Autodesk Fusion 360 part; units mm, degrees
(part 4 of 4)
extrude "Extrude2" cut sketch "IronHandPCBPlate" along normal blind 1.2 contours L457 L479 L536 L538 L540 L541 L542 L543 bodies 1
extrude "Extrude3" add sketch "Sketch3" along normal blind 1 separate body contours A4 | L212 L490 L491 L492 L495 | L212 L486 L492 L496 | L212 L484 L485 L486 L489 L495 L496 | L212 L483 L484 L487 L489 L494 L495 | L212 L467 L486 L492 | L212 L213 L214 L218 L464 L466 L467 L468 L477 L478 L479 L481 L490 L491 L492 L499 L518 | L486 L492 L496 L511 | L485 L486 L496 L497 L505 | L212 L213 L487 L490 L494 | L482 L483 L484 L485 L502 | L467 L486 L492 L511 | L492 L493 L497 L498 L505 L509 L511 | L483 L487 L494 L497 L503 | L213 L487 L490 L493 L494 L497 L498 L503 | L467 L492 L509 L511 | L482 L497 L502 L505 L517 | L493 L497 L498 L505 L509 L517 | L493 L498 L501 L505 L509 L515 | L467 L501 L508 L509 L515 | L482 L497 L502 L503 L517 | L493 L497 L498 L503 L517 | L493 L498 L505 L509 L510 L515 | L213 L493 L498 L499 L500 L503 L504 L506 L507 | L501 L505 L513 L515 | L467 L501 L508 L513 L514 L515 | L493 L498 L503 L504 L510 L513 L515 L516 | L505 L510 L513 L515 | L213 L466 L467 L500 L512 L518 | L501 L505 L507 L513 | L467 L501 L507 L508 L513 | L510 L513 L515 L516 | L504 L505 L507 L510 L513 | L214 L466 L468 L477 L518 L519 L520 L521 | L500 L501 L504 L506 L507 | L467 L501 L507 L512 | A249 | A458 makes body 2
extrude "Extrude4" add sketch "Sketch3" along normal blind 5.5 contours L212 L490 L491 L492 L495 | L212 L486 L492 L496 | L212 L484 L485 L486 L489 L495 L496 | L212 L483 L484 L487 L489 L494 L495 | L486 L492 L496 L511 | L485 L486 L496 L497 L505 | L212 L213 L487 L490 L494 | L492 L493 L497 L498 L505 L509 L511 | L483 L487 L494 L497 L503 | L213 L487 L490 L493 L494 L497 L498 L503 | L467 L492 L509 L511 | L482 L497 L502 L505 L517 | L493 L497 L498 L505 L509 L517 | L493 L498 L501 L505 L509 L515 | L467 L501 L508 L509 L515 | L482 L497 L502 L503 L517 | L493 L497 L498 L503 L517 | L493 L498 L505 L509 L510 L515 | L213 L493 L498 L499 L500 L503 L504 L506 L507 | L501 L505 L513 L515 | L467 L501 L508 L513 L514 L515 | L493 L498 L503 L504 L510 L513 L515 L516 | L505 L510 L513 L515 | L501 L505 L507 L513 | L467 L501 L507 L508 L513 | L510 L513 L515 L516 | L504 L505 L507 L510 L513 | L500 L501 L504 L506 L507 | L467 L501 L507 L512 bodies 2
extrude "Extrude5" cut sketch "Sketch3" against normal blind 3 from surface at 5.5 contours L212 L484 L485 L486 L489 L495 L496 | L212 L483 L484 L487 L489 L494 L495 | L485 L486 L496 L497 L505 | L483 L487 L494 L497 L503 | L482 L497 L502 L505 L517 | L482 L497 L502 L503 L517 bodies 2
extrude "Extrude8" add sketch "Sketch3" along normal blind 4.5 contours L493 L498 L501 L505 L509 L515 | L467 L501 L508 L509 L515 | L493 L498 L505 L509 L510 L515 | L501 L505 L513 L515 | L467 L501 L508 L513 L514 L515 | L493 L498 L503 L504 L510 L513 L515 L516 | L505 L510 L513 L515 | L501 L505 L507 L513 | L467 L501 L507 L508 L513 | L510 L513 L515 L516 | L504 L505 L507 L510 L513 bodies 2
sketch "Sketch4" plane through (0, 0, 7.5) normal (0, 0, 1) x (-1, 0, 0)
  line L0 (37.7668, 220.6) -> (37.7667, 165.6443)
  line L1 (37.7667, 165.6443) -> (61.9431, 165.6443)
  line L2 (61.9431, 165.6443) -> (61.9431, 201.6)
  line L3 (60.9431, 166.6443) -> (38.7668, 166.6443)
  line L4 (38.7667, 166.6443) -> (38.7667, 201.6)
  line L5 (38.7667, 201.6) -> (60.9431, 201.6)
  line L6 (60.9431, 201.6) -> (60.9431, 166.6443)
  line L7 (67.9431, 220.6) -> (37.7668, 220.6)
  line L8 (61.9431, 201.6) -> (67.9431, 201.6)
  line L9 (67.9431, 201.6) -> (67.9431, 220.6)
  line L10 (67.9431, 231.6) -> (64.9431, 231.6) construction
  line L11 (64.9431, 231.6) -> (64.9431, 229.1)
  line L12 (64.9431, 229.1) -> (67.9431, 229.1)
  line L13 (67.9431, 229.1) -> (67.9431, 231.6) construction
  line L14 (67.9431, 229.1) -> (64.9431, 229.1)
  line L15 (64.9431, 229.1) -> (64.9431, 226.1)
  line L16 (64.9431, 226.1) -> (67.9431, 226.1)
  line L17 (67.9431, 226.1) -> (67.9431, 229.1)
  line L18 (38.7667, 166.6443) -> (38.7667, 201.6)
  line L19 (38.7667, 201.6) -> (60.9431, 201.6)
  line L20 (60.9431, 201.6) -> (60.9431, 166.6443)
  line L21 (60.9431, 166.6443) -> (38.7668, 166.6443)
  point P0 (67.9431, 231.6)
  point P1 (67.9431, 231.6)
  dimension "d76" = 3
  dimension "d77" = 2.5
  dimension "d100" = 3
  dimension "d101" = 3
  constraint horizontal L3
  constraint vertical L4
  constraint horizontal L5
  constraint vertical L6
  constraint horizontal L10
  constraint vertical L11
  constraint horizontal L12
  constraint vertical L13
  constraint coincident P1 P0
  constraint horizontal L14
  constraint vertical L15
  constraint horizontal L16
  constraint vertical L17
  measures "d76" distance of P1 L10.end
  measures "d77" distance of P1 L12.end
  measures "d100" distance of L12.end L11.end
  measures "d101" distance of L12.end L16.end
extrude "Extrude6" add sketch "Sketch4" against normal blind 3 separate body contours L3 L4 L5 L6 L18 L19 L20 L21 makes body 3
extrude "Extrude7" cut sketch "Sketch3" along normal blind 2.5 contours L482 L483 L484 L485 L502 | L482 L497 L502 L505 L517 | L493 L497 L498 L505 L509 L517 | L493 L498 L501 L505 L509 L515 | L467 L501 L508 L509 L515 | L493 L498 L505 L509 L510 L515 | L501 L505 L513 L515 | L467 L501 L508 L513 L514 L515 | L505 L510 L513 L515 | L501 L505 L507 L513 | L467 L501 L507 L508 L513 | L504 L505 L507 L510 L513 bodies 2
extrude "Extrude9" cut sketch "Sketch3" along normal blind 3.5 contours L501 L505 L513 L515 | L467 L501 L508 L513 L514 L515 | L505 L510 L513 L515 bodies 2
extrude "Extrude10" add sketch "Sketch4" against normal up to surface (2.5 mm away) from surface at -5 contours L12 L14 L15 L16 L17 bodies 2
sketch "Sketch5" plane through (-67.9431, 0, 0) normal (-1, 0, 0) x (0, -1, 0)
  line L0 (218.7407, 5.5) -> (218.7407, 4.5)
  line L1 (218.7407, 4.5) -> (219.6, 4.5)
  line L2 (219.6, 4.5) -> (219.6, 2)
  line L3 (229.1, 2) -> (231.6, 2)
  line L4 (226.1, 0) -> (229.1, 0)
  line L5 (231.6, 3) -> (220.6, 3)
  line L6 (220.6, 3) -> (220.6, 7.5)
  line L7 (220.6, 7.5) -> (201.6, 7.5)
  line L8 (201.6, 7.5) -> (201.6, 3)
  line L9 (201.6, 3) -> (156.6443, 3)
  line L10 (156.6443, 3) -> (156.6443, 2)
  line L11 (156.6443, 2) -> (202.6, 2)
  line L12 (202.6, 2) -> (202.6, 4.5)
  line L13 (202.6, 4.5) -> (203.6, 4.5)
  line L14 (203.6, 4.5) -> (203.6, 5.5)
  line L15 (203.6, 5.5) -> (218.7407, 5.5)
  line L16 (202.6, 6.5) -> (202.6, 4.2) construction
  line L17 (202.6, 4.2) -> (201.6, 4.2)
  line L18 (201.6, 4.2) -> (201.6, 7.5)
  line L19 (201.6, 7.5) -> (202.6, 7.5)
  line L20 (202.6, 7.5) -> (202.6, 4.2) construction
  line L21 (202.6, 7.5) -> (202.6, 6.5)
  line L22 (202.6, 7.5) -> (220.6, 7.5)
  line L23 (220.6, 7.5) -> (220.6, 6.5)
  line L24 (220.6, 7.5) -> (220.6, 3.7)
  line L25 (202.6, 4.2) -> (202.6, 4.5)
  line L26 (202.6, 4.5) -> (203.6, 4.5)
  line L27 (203.6, 4.5) -> (203.6, 5.5)
  line L28 (203.6, 5.5) -> (218.7407, 5.5)
  line L29 (218.7407, 5.5) -> (218.7407, 4.5)
  line L30 (218.7407, 4.5) -> (219.6, 4.5)
  line L31 (219.6, 4.5) -> (219.6, 3.6999)
  line L32 (219.6, 3.6999) -> (220.6, 3.7)
  line L33 (231.6, 2) -> (231.6, 3)
  line L34 (219.6, 2) -> (226.1, 2)
  line L35 (226.1, 2) -> (226.1, 0)
  line L36 (219.6, 2) -> (214.35, 2) construction
  line L37 (214.35, 2) -> (214.35, 1) construction
  line L38 (214.35, 1) -> (219.6, 1) construction
  line L39 (219.6, 1) -> (219.6, 2) construction
  circle A0 centre (214.35, 2) radius 3.55
  line L40 (229.1, 0) -> (229.1, 2)
  dimension "d81" = 2.3
  dimension "d102" = 5.25
  dimension "d106" = 1
  dimension "d107" = 7.1
  constraint perpendicular L7 L16
  constraint horizontal L17
  constraint vertical L18
  constraint horizontal L19
  constraint vertical L20
  constraint coincident L7.end L8.start
  constraint coincident L6.end L7.start
  constraint perpendicular L17 L24
  constraint coincident L12.end L13.start
  constraint coincident L13.end L14.start
  constraint coincident L14.end L15.start
  constraint coincident L0.start L15.end
  constraint coincident L0.end L1.start
  constraint coincident L1.end L2.start
  constraint coincident L2 L31.end
  constraint horizontal L36
  constraint vertical L37
  constraint horizontal L38
  constraint vertical L39
  constraint coincident L2.end L34.start
  constraint coincident L36.end L37.start
  constraint coincident L19.end L20.start
  measures "d81" distance of L16.start L16.end
  measures "d102" distance of L2.end L36.end
  measures "d106" distance of L2.end L38.end
  measures "d107" diameter of A0
extrude "Extrude11" add sketch "Sketch5" along normal blind 4 contours L0 L1 L2 L6 L7 L8 L12 L13 L14 L15 L17 L18 L19 L22 L23 L24 L25 L26 L27 L28 L29 L30 L31 L32 A0 | L15 L28 A0 | L2 L3 L4 L5 L6 L32 L33 L34 L35 L40 | L8 L9 L10 L11 L12 L17 picked at (214.2838, 5.5148) bodies 2
sketch "Sketch6" plane through (0, 0, 5.5) normal (0, 0, -1) x (1, 0, 0)
  line L0 (-71.9431, 203.6) -> (-43.2667, 203.6)
  line L1 (-43.2668, 203.6) -> (-43.2668, 218.7407)
  line L2 (-43.2668, 218.7407) -> (-71.9431, 218.7407)
  line L3 (-71.9431, 218.7407) -> (-71.9431, 203.6)
  line L4 (-71.9431, 219.6) -> (-69.9431, 219.6)
  line L5 (-69.9431, 219.6) -> (-69.9431, 202.5572)
  line L6 (-69.9431, 202.5572) -> (-71.9431, 202.5572)
  line L7 (-71.9431, 202.5572) -> (-71.9431, 219.6)
  point P0 (-71.9431, 219.6)
  point P1 (-71.9431, 202.6)
  dimension "d84" = 2
  constraint horizontal L4
  constraint vertical L5
  constraint horizontal L6
  constraint vertical L7
  constraint coincident P0 L4.start
  measures "d84" distance of P0 L4.end
extrude "Extrude12" add sketch "Sketch6" along normal up to surface (3.5 mm away) contours L0 L2 L3 L5 L7 | L0 L5 L6 L7 | L2 L4 L5 L7 bodies 2
sketch "Sketch7" plane through (0, 0, 3) normal (0, 0, 1) x (-1, 0, 0)
  line L0 (71.9431, 201.6) -> (61.9431, 201.6)
  line L1 (61.9431, 201.6) -> (61.9431, 165.6443)
  line L2 (61.9431, 165.6443) -> (37.7667, 165.6443)
  line L3 (37.7667, 165.6443) -> (37.7668, 220.6)
  line L4 (37.7668, 220.6) -> (71.9431, 220.6)
  line L5 (22.0127, 228.6) -> (21.9431, 228.6)
  line L6 (21.9431, 228.6) -> (21.9431, 218.6)
  line L7 (21.9431, 218.6) -> (36.4431, 218.6)
  line L8 (36.4431, 218.6) -> (36.4431, 156.6443)
  line L9 (36.4431, 156.6443) -> (71.9431, 156.6443)
  line L10 (71.9431, 220.6) -> (71.9431, 231.6)
  line L11 (71.9431, 156.6443) -> (71.9431, 201.6)
  line L12 (71.9431, 231.6) -> (69.9431, 231.6)
  line L13 (69.9431, 231.6) -> (69.9431, 225.5978)
  line L14 (69.9431, 225.5978) -> (71.9431, 225.5978)
  line L15 (71.9431, 225.5978) -> (71.9431, 231.6)
  line L16 (71.9431, 231.6) -> (22.0127, 231.6)
  line L17 (22.0127, 231.6) -> (22.0127, 228.6)
  point P0 (27.4668, 224.6)
  point P1 (62.9431, 161.6443)
  point P2 (42.9431, 161.6443)
  dimension "d94" = 2
  constraint horizontal L12
  constraint vertical L13
  constraint horizontal L14
  constraint vertical L15
  constraint coincident L10.end L12.start
  measures "d94" distance of L10.end L12.end
hole "Hole1" at (-27.4668, -224.6, 3) at (-42.9431, -161.6443, 3) at (-62.9431, -161.6443, 3) direction (0, 0, -1) diameter 3.4 depth 4 tip angle 180 countersink diameter 6.3 countersink angle 90 bodies 1 2
extrude "Extrude13" cut sketch "Sketch7" against normal blind 2 from surface at -1 contours L10 L12 L13 L14 L15 L16 bodies 1 2
extrude "Extrude14" cut sketch "Sketch5" along normal blind 4 contours L15 L28 A0 | L15 L28 A0 bodies 2
ref_plane "WorkPlane1" through (0, -2.5, 0) normal (0, 1, 0) x (0, 0, 1)
split "Split1" by plane through (0, -2.5, 0) normal (0, 1, 0) bodies 1 makes body 4 at (47.9166, 26.0099, 2)
sketch "Sketch8" plane through (0, 0, 7.5) normal (0, 0, 1) x (-1, 0, 0)
  line L0 (38.7667, 166.6443) -> (38.7667, 201.6)
  line L1 (38.7667, 201.6) -> (60.9431, 201.6)
  line L2 (60.9431, 201.6) -> (60.9431, 166.6443)
  line L3 (60.9431, 166.6443) -> (38.7668, 166.6443)
  line L4 (37.7668, 220.6) -> (37.7667, 165.6443)
  line L5 (37.7667, 165.6443) -> (61.9431, 165.6443)
  line L6 (61.9431, 165.6443) -> (61.9431, 201.6)
  line L7 (61.9431, 201.6) -> (71.9431, 201.6)
  line L8 (71.9431, 201.6) -> (71.9431, 220.6)
  line L9 (71.9431, 220.6) -> (37.7668, 220.6)
  line L10 (71.9431, 201.6) -> (61.9431, 201.6)
  line L11 (61.9431, 201.6) -> (61.9431, 202.6)
  line L12 (61.9431, 202.6) -> (71.9431, 202.6)
  line L13 (71.9431, 202.6) -> (71.9431, 201.6)
  line L14 (71.9431, 220.6) -> (37.7668, 220.6)
  line L15 (37.7668, 220.6) -> (37.7668, 219.6)
  line L16 (37.7668, 219.6) -> (71.9431, 219.6)
  line L17 (71.9431, 219.6) -> (71.9431, 220.6)
  line L18 (37.7668, 219.6) -> (38.7668, 219.6)
  line L19 (38.7668, 219.6) -> (38.7668, 202.6)
  line L20 (38.7668, 202.6) -> (37.7668, 202.6)
  line L21 (37.7668, 202.6) -> (37.7668, 219.6)
  dimension "d110" = 1
  dimension "d111" = 1
  dimension "d112" = 1
  dimension "d113" = 17
  constraint horizontal L10
  constraint vertical L11
  constraint horizontal L12
  constraint vertical L13
  constraint coincident L7.end L8.start
  constraint horizontal L14
  constraint vertical L15
  constraint horizontal L16
  constraint vertical L17
  constraint coincident L8.end L9.start
  constraint horizontal L18
  constraint vertical L19
  constraint horizontal L20
  constraint vertical L21
  measures "d110" distance of L7.end L12.end
  measures "d111" distance of L8.end L16.end
  measures "d112" distance of L15.end L18.end
  measures "d113" distance of L15.end L20.end
extrude "Extrude15" cut sketch "Sketch8" against normal blind 1 contours L4 L8 L9 L14 L15 L16 L17 L18 | L4 L16 L18 L19 L20 L21 | L7 L8 L10 L11 L12 L13 bodies 2
combine "Combine1" operation add target body 4 tool bodies 1
hidden bodies 2 3
